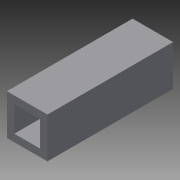
# Autodesk Inventor part: arm-seg1
Saved by Autodesk Inventor 2016 (Build 200138000, 138)
## iProperties
Created: 2015-10-13
Part Number: arm-seg1
Material: Generic
Document SubType Name: Modeling
Designer: eedoga
Density: 1 g/cm^3
Appearance: Default
Author: eedoga
Autodesk Inventor part; units mm, degrees
ref_plane "YZ Plane" through (0, 0, 0) normal (1, 0, 0) x (0, 1, 0)
ref_plane "XZ Plane" through (0, 0, 0) normal (0, 1, 0) x (-1, 0, 0)
ref_plane "XY Plane" through (0, 0, 0) normal (0, 0, 1) x (1, 0, 0)
sketch "Sketch1" plane through (0, 0, 0) normal (0, 0, 1) x (1, 0, 0)
  line L0 (-5, 12.5) -> (5, 12.5) projected
  line L1 (5, 12.5) -> (5, 2.5) projected
  line L2 (5, 2.5) -> (-5, 2.5) projected
  line L3 (-5, 2.5) -> (-5, 12.5) projected
  line L4 (-6.5, 1) -> (-6.5, 14) projected
  line L5 (6.5, 1) -> (-6.5, 1) projected
  line L6 (6.5, 14) -> (6.5, 1) projected
  line L7 (-6.5, 14) -> (6.5, 14) projected
  line L8 (-5, 2.5) -> (5, 2.5)
  line L9 (5, 2.5) -> (5, 12.5)
  line L10 (5, 12.5) -> (-5, 12.5)
  line L11 (-5, 12.5) -> (-5, 2.5)
  line L12 (4.1303, 3.3697) -> (-4.1303, 3.3697)
  line L13 (-4.1303, 3.3697) -> (-4.1303, 11.6303)
  line L14 (-4.1303, 11.6303) -> (4.1303, 11.6303)
  line L15 (4.1303, 11.6303) -> (4.1303, 3.3697)
  line L16 (-4.1303, 3.3697) -> (4.1303, 11.6303) construction
  point P0 (0, 0)
  point P1 (0, 7.5)
  constraints: 18 end point, 4 parallel, 2 horizontal, 2 perpendicular, 1 midpoint
extrude "Extrusion1" add sketch "Sketch1" along normal blind 30 contours L0 L1 L2 L3
sketch "Sketch2" plane through (0, 0, 30) normal (0, 0, 1) x (1, 0, 0)
  line L0 (-5, 2.5) -> (5, 2.5) projected
  line L1 (5, 2.5) -> (5, 12.5) projected
  line L2 (5, 12.5) -> (-5, 12.5) projected
  line L3 (-5, 12.5) -> (-5, 2.5) projected
  line L4 (3.175, 4.325) -> (-3.175, 4.325)
  line L5 (-3.175, 4.325) -> (-3.175, 10.675)
  line L6 (-3.175, 10.675) -> (3.175, 10.675)
  line L7 (3.175, 10.675) -> (3.175, 4.325)
  line L8 (-3.175, 4.325) -> (3.175, 10.675) construction
  point P0 (0, 0)
  point P1 (0, 7.5)
  constraints: 10 end point, 2 parallel, 1 horizontal, 1 midpoint, 1 perpendicular
extrude "Extrusion2" add sketch "Sketch2" along normal blind 1
body "Solid1"
